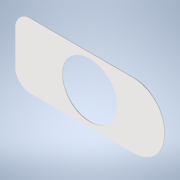
# Autodesk Inventor part: Bodenplatte-Holz
Saved by Autodesk Inventor 2020.3 (Build 243373010, 373A)
## iProperties
Created: 2021-01-31
Part Number: Bodenplatte-Holz
Material: Generisch
Document SubType Name: Modeling
Designer: Stefan
Density: 1 g/cm^3
Appearance: Vorgabe
Author: Stefan
Autodesk Inventor part; units mm, degrees
ref_plane "YZ Plane" through (0, 0, 0) normal (1, 0, 0) x (0, 1, 0)
ref_plane "XZ Plane" through (0, 0, 0) normal (0, 1, 0) x (-1, 0, 0)
ref_plane "XY Plane" through (0, 0, 0) normal (0, 0, 1) x (1, 0, 0)
sketch "Skizze2" plane through (0, 0, 0) normal (0, 0, 1) x (1, 0, 0)
  line L0 (-775, 425) -> (575, 425)
  line L1 (975, 25) -> (975, -25)
  line L2 (575, -425) -> (-775, -425)
  line L3 (-975, -225) -> (-975, 225)
  arc A0 (975, 25) -> (575, 425) centre (575, 25) ccw
  arc A1 (575, -425) -> (975, -25) centre (575, -25) ccw
  arc A2 (-775, 425) -> (-975, 225) centre (-775, 225) ccw
  arc A3 (-975, -225) -> (-775, -425) centre (-775, -225) ccw
  circle A4 centre (0, 0) radius 360
  point P0 (975, -425)
  point P1 (975, 425)
  point P2 (-975, -425)
  dimension "d0" = 850
  dimension "d1" = 1950
  dimension "d2" = 400
  dimension "d3" = 200
  dimension "d4" = 720
  dimension "d5" = 975
  dimension "d6" = 425
  constraints: 8 end point, 8 point on circle, 8 tangent, 6 point on line, 5 centre point, 2 equal radius, 2 parallel, 1 coincident, 1 horizontal, 1 perpendicular
  measures "d0" distance of point (975, 425) point (975, -425)
  measures "d1" distance of point (975, -425) point (-975, -425)
  measures "d2" radius of A0
  measures "d3" radius of A2
  measures "d4" diameter of A4
  measures "d5" distance from line of L1 A4.centre
  measures "d6" distance from line of L0 A4.centre
extrude "Extrusion1" add sketch "Skizze2" along normal blind 10
